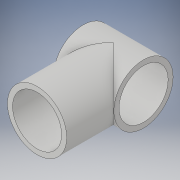
# Autodesk Inventor part: Slip Tee 1 Inch
Saved by Autodesk Inventor 2018 (Build 220112000, 112)
## iProperties
Created: 2018-01-16
Part Number: Slip Tee 1 Inch
Material: Generic
Document SubType Name: Modeling
Designer: owner
Density: 1 g/cm^3
Appearance: Default
Author: owner
Autodesk Inventor part; units mm, degrees
ref_plane "YZ Plane" through (0, 0, 0) normal (1, 0, 0) x (0, 1, 0)
ref_plane "XZ Plane" through (0, 0, 0) normal (0, 1, 0) x (-1, 0, 0)
sketch "Sketch1" plane through (0, 0, 0) normal (0, 0, 1) x (1, 0, 0)
  circle A0 centre (0, 0) radius 20.2565
  dimension "d1" = 40.513
  constraints: 1 centre point
  measures "d1" diameter of A0
sketch "Sketch2" plane through (0, 0, 0) normal (1, 0, 0) x (0, 1, 0)
  line L0 (0, 0) -> (27.2274, 0)
  line L1 (27.2274, 0) -> (27.2274, -51.0956)
  line L2 (27.2274, -51.0956) -> (0, -51.0956)
  line L3 (0, -51.0956) -> (0, 0)
  constraints: 8 end point, 2 parallel, 1 horizontal, 1 perpendicular
ref_plane "Work Plane2" through (20.6375, 27.2274, 0) normal (-1, 0, 0) x (0, 0, -1)
ref_plane "Work Plane1" through (0, 27.2274, 0) normal (-1, 0, 0) x (0, 0, -1)
extrude "Extrusion1" add sketch "Sketch1" against normal blind 52.0573
sketch "Sketch3" plane through (0, 0, 0) normal (0, 0, 1) x (1, 0, 0)
  circle A0 centre (0, 0) radius 16.7767
  dimension "d5" = 33.5534
  constraints: 1 centre point, 1 coincident
  measures "d5" diameter of A0
sketch "Sketch4" plane through (20.6375, 27.2274, 0) normal (-1, 0, 0) x (0, 0, -1)
  line L0 (52.0573, 6.9709) -> (52.0573, 47.4839) projected
  circle A0 centre (52.0573, 27.2274) radius 20.2565
  point P0 (0, 27.2274)
  constraints: 1 centre point
sketch "Sketch5" plane through (20.6375, 27.2274, 0) normal (-1, 0, 0) x (0, 0, -1)
  circle A0 centre (52.1379, 27.2274) radius 16.7767
  point P0 (0, 27.2274)
  dimension "d10" = 33.5534
  constraints: 1 centre point
  measures "d10" diameter of A0
extrude "Extrusion2" add sketch "Sketch4" along normal blind 41.275
extrude "Extrusion3" cut sketch "Sketch5" along normal through all
extrude "Extrusion4" cut sketch "Sketch3" against normal blind 31.9024
body "Solid1"
